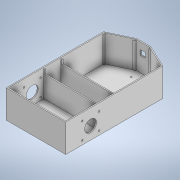
# Autodesk Inventor part: Robot
Saved by Autodesk Inventor 2020 (Build 240168000, 168)
## iProperties
Created: 2020-03-26
Part Number: Robot
Material: Generic
Document SubType Name: Modeling
Designer: Ondra
Density: 1 g/cm^3
Appearance: Default
Author: Ondra
Autodesk Inventor part; units mm, degrees
ref_plane "YZ Plane" through (0, 0, 0) normal (1, 0, 0) x (0, 1, 0)
ref_plane "XZ Plane" through (0, 0, 0) normal (0, 1, 0) x (-1, 0, 0)
ref_plane "XY Plane" through (0, 0, 0) normal (0, 0, 1) x (1, 0, 0)
sketch "Sketch1" plane through (0, 0, 0) normal (0, 1, 0) x (-1, 0, 0)
  line L0 (0, 0) -> (110, 0)
  line L1 (110, 0) -> (110, -180)
  line L2 (0, -180) -> (0, 0)
  line L3 (67.5, -200) -> (42.5, -200)
  line L4 (67.5, -200) -> (110, -180)
  line L5 (42.5, -200) -> (0, -180)
  dimension "d2" = 180
  dimension "d38" = 25
  constraints: 12 end point, 1 horizontal, 1 parallel, 1 perpendicular
  measures "d2" distance of L0.end L1.end
  measures "d38" distance of L3.start L3.end
extrude "Extrusion1" add sketch "Sketch1" along normal blind 2
sketch "Sketch2" plane through (0, 2, 0) normal (0, 1, 0) x (1, 0, 0)
  line L0 (0, 180) -> (-110, 180) projected
  line L1 (-110, 180) -> (-110, 0) projected
  line L2 (0, 180) -> (-110, 180)
  line L3 (-110, 180) -> (-110, 0)
  line L4 (-110, 0) -> (0, 0)
  line L5 (0, 0) -> (0, 180)
  line L6 (0, 0) -> (0, 180) projected
  line L7 (-110, 0) -> (0, 0) projected
  line L8 (-2, 2) -> (-108, 2)
  line L9 (-108, 2) -> (-108, 178)
  line L10 (-108, 178) -> (-2, 178)
  line L11 (-2, 178) -> (-2, 2)
  constraints: 16 end point, 4 parallel, 2 horizontal, 2 perpendicular
extrude "Extrusion2" add sketch "Sketch2" along normal blind 50
sketch "Sketch3" plane through (-108, 2, -2) normal (1, 0, 0) x (0, 0, -1)
  line L0 (0, 50) -> (176, 50) projected
  line L1 (65, 40) -> (65, 0)
  line L2 (176, 0) -> (0, 0) projected
  line L3 (67, 40) -> (67, 0)
  line L4 (67, 0) -> (65, 0)
  line L5 (97, 40) -> (97, 0)
  line L6 (97, 0) -> (99, 0)
  line L7 (99, 0) -> (99, 40)
  line L8 (65, 40) -> (67, 40)
  line L9 (99, 40) -> (97, 40)
  point P0 (-2, -2)
  point P1 (67, 0)
  constraints: 16 end point, 5 point on line, 4 perpendicular
extrude "Extrusion3" add sketch "Sketch3" along normal up to next
sketch "Sketch4" plane through (0, 2, 0) normal (0, 1, 0) x (1, 0, 0)
  line L0 (-108, 69) -> (-2, 69) projected
  line L1 (-90, 69) -> (-90, 99)
  line L2 (-108, 99) -> (-2, 99) projected
  line L3 (-2, 69) -> (-2, 99) projected
  line L4 (-20, 69) -> (-20, 99)
  line L5 (-20, 99) -> (-90, 99)
  line L6 (-90, 69) -> (-20, 69)
  point P0 (0, 0)
  constraints: 8 end point, 2 point on line, 1 collinear, 1 perpendicular
extrude "Extrusion4" cut sketch "Sketch4" against normal up to next contours L1 L2 L4 L0
sketch "Sketch5" plane through (-108, 2, -178) normal (1, 0, 0) x (0, 0, -1)
  line L0 (-111, 0) -> (-111, 40) projected
  line L1 (-111, 0) -> (-176, 0) projected
  circle A0 centre (-132, 21) radius 11
  circle A1 centre (-147.5, 36.5) radius 1.5
  circle A2 centre (-116.5, 36.5) radius 1.5
  circle A3 centre (-147.5, 36.5) radius 1.5
  circle A4 centre (-147.5, 5.5) radius 1.5
  circle A5 centre (-116.5, 5.5) radius 1.5
  point P0 (-178, -2)
  constraints: 6 centre point
extrude "Extrusion5" cut sketch "Sketch5" along normal through all both and the other way through all
sketch "Sketch6" plane through (-108, 2, -178) normal (0, 0, 1) x (1, 0, 0)
  line L0 (106, 0) -> (106, 50) projected
  line L1 (106, 50) -> (0, 50)
  line L2 (0, 50) -> (0, 0)
  line L3 (0, 0) -> (106, 0)
  line L4 (106, 0) -> (106, 50)
  point P0 (108, -2)
  constraints: 8 end point, 2 parallel, 1 horizontal, 1 perpendicular
extrude "Extrusion6" cut sketch "Sketch6" against normal up to next
sketch "Sketch7" plane through (0, 2, 0) normal (0, 1, 0) x (1, 0, 0)
  line L0 (-67.5, 200) -> (-110, 180) projected
  line L1 (-110, 180) -> (-67.5, 200)
  line L2 (-67.5, 200) -> (-42.5, 200)
  line L3 (0, 180) -> (-42.5, 200) projected
  line L4 (-42.5, 200) -> (0, 180)
  line L5 (-67.5, 198) -> (-42.5, 198)
  line L6 (-99.9511, 182.7289) -> (-67.5, 198)
  line L7 (-99.9511, 182.7289) -> (-108, 178.9412)
  line L8 (-108, 180) -> (-108, 101) projected
  line L9 (-108, 180) -> (-110, 180)
  line L10 (-21.25, 188) -> (-42.5, 198)
  line L11 (-21.25, 188) -> (-2, 178.9412)
  line L12 (-2, 101) -> (-2, 180) projected
  line L13 (-2, 180) -> (0, 180)
  line L14 (0, 180) -> (-42.5, 200)
  line L15 (-42.5, 200) -> (-67.5, 200) projected
  line L16 (-42.5, 200) -> (-67.5, 200)
  line L17 (-110, 180) -> (-110, 0) projected
  line L18 (-67.5, 200) -> (-110, 180)
  point P0 (0, 0)
  constraints: 26 end point, 4 point on line, 3 collinear, 1 horizontal, 1 parallel, 1 perpendicular
extrude "Extrusion7" add sketch "Sketch7" along normal up to surface (50 mm away)
sketch "Sketch8" plane through (-42.5, 0, -200) normal (0, 0, -1) x (-1, 0, 0)
  line L0 (0, 0) -> (25, 0) projected
  line L1 (8, 39.5) -> (17, 39.5)
  line L2 (17, 39.5) -> (17, 30.5)
  line L3 (17, 30.5) -> (8, 30.5)
  line L4 (8, 30.5) -> (8, 39.5)
  line L5 (8, 39.5) -> (17, 30.5) construction
  line L6 (17, 39.5) -> (8, 30.5) construction
  point P0 (-42.5, 0)
  dimension "d48" = 9
  dimension "d49" = 9
  constraints: 12 end point, 2 parallel, 1 horizontal, 1 perpendicular
  measures "d48" distance of L2.end L3.end
  measures "d49" distance of L1.end L2.end
extrude "Extrusion8" cut sketch "Sketch8" against normal blind 2
sketch "Sketch9" plane through (0, 2, 0) normal (0, 1, 0) x (1, 0, 0)
  line L0 (-108, 2) -> (-108, 178.9412) projected
  line L1 (-108, 2) -> (-106, 2)
  line L2 (-106, 2) -> (-106, 4)
  line L3 (-106, 4) -> (-108, 4)
  line L4 (-108, 4) -> (-108, 2)
  line L5 (-2, 2) -> (-108, 2) projected
  line L6 (-2, 2) -> (-4, 2)
  line L7 (-4, 2) -> (-4, 4)
  line L8 (-4, 4) -> (-2, 4)
  line L9 (-2, 4) -> (-2, 2)
  line L10 (-67.5, 198) -> (-108, 178.9412) projected
  line L11 (-106, 178.9412) -> (-106, 176.9412)
  line L12 (-106, 176.9412) -> (-108, 176.9412)
  line L13 (-108, 176.9412) -> (-108, 178.9412)
  line L14 (-106, 178.9412) -> (-106, 179.8824)
  line L15 (-108, 178.9412) -> (-108, 101) projected
  line L16 (-108, 178.9412) -> (-106, 179.8824)
  line L17 (-2, 178.9412) -> (-2, 2) projected
  line L18 (-4, 178.9412) -> (-4, 176.9412)
  line L19 (-4, 176.9412) -> (-2, 176.9412)
  line L20 (-2, 176.9412) -> (-2, 178.9412)
  line L21 (-4, 178.9412) -> (-4, 179.8824)
  line L22 (-2, 178.9412) -> (-42.5, 198) projected
  line L23 (-4, 179.8824) -> (-2, 178.9412)
  line L24 (-4, 179.8824) -> (-2, 178.9412)
  line L25 (-67.5, 198) -> (-108, 178.9412) projected
  line L26 (-67.5, 198) -> (-67.5, 196)
  line L27 (-67.5, 196) -> (-71.75, 196)
  line L28 (-42.5, 198) -> (-67.5, 198) projected
  line L29 (-42.5, 198) -> (-42.5, 196)
  line L30 (-42.5, 196) -> (-38.25, 196)
  line L31 (-42.5, 198) -> (-38.25, 196)
  line L32 (-71.75, 196) -> (-67.5, 198)
  line L33 (-55, 2) -> (-53, 2)
  line L34 (-53, 2) -> (-53, 4)
  line L35 (-53, 4) -> (-57, 4)
  line L36 (-57, 4) -> (-57, 2)
  line L37 (-57, 2) -> (-55, 2)
  point P0 (0, 0)
  constraints: 60 end point, 7 point on line, 6 parallel, 5 perpendicular, 3 collinear, 3 vertical, 2 horizontal, 1 midpoint
extrude "Extrusion9" add sketch "Sketch9" along normal blind 48 contours L0 L3 L2 L1 | L36 L35 L34 L5 | L0 L10 L14 L11 L12 | L7 L8 L9 L5 | L10 L26 L27 | L22 L30 L29 | L19 L18 L21 L22 L17
sketch "Sketch10" plane through (-108, 42, -101) normal (0, 1, 0) x (1, 0, 0)
  line L0 (0, 0) -> (106, 0) projected
  line L1 (0, -2) -> (106, -2) projected
  line L2 (106, 0) -> (104, 0)
  line L3 (104, 0) -> (104, -2)
  line L4 (104, -2) -> (106, -2)
  line L5 (106, -2) -> (106, 0)
  line L6 (106, -32) -> (106, -34) projected
  line L7 (106, -32) -> (104, -32)
  line L8 (104, -32) -> (104, -34)
  line L9 (104, -34) -> (106, -34)
  line L10 (106, -34) -> (106, -32)
  line L11 (106, -34) -> (0, -34) projected
  line L12 (0, -32) -> (18, -32) projected
  line L13 (0, -34) -> (2, -34)
  line L14 (2, -34) -> (2, -32)
  line L15 (2, -32) -> (0, -32)
  line L16 (0, -32) -> (0, -34)
  line L17 (0, -2) -> (0, 0) projected
  line L18 (0, 0) -> (2, 0)
  line L19 (2, 0) -> (2, -2)
  line L20 (2, -2) -> (0, -2)
  line L21 (0, -2) -> (0, 0)
  point P0 (108, -101)
  point P1 (2, -34)
  point P2 (2, -2)
  point P3 (2, 0)
  constraints: 32 end point, 8 parallel, 4 horizontal, 4 perpendicular, 3 point on line
extrude "Extrusion10" add sketch "Sketch10" along normal blind 8 contours L0 L19 L1 L17 | L0 L5 L1 L3 | L11 L16 L12 L14 | L6 L9 L8 L7
sketch "Sketch12" plane through (0, 2, 0) normal (0, 1, 0) x (1, 0, 0)
  line L0 (-106, 99) -> (-4, 99) projected
  line L1 (-55, 99) -> (-100, 99)
  line L2 (-100, 99) -> (-100, 69)
  line L3 (-108, 101) -> (-2, 101) projected
  line L4 (-100, 99) -> (-70, 99) construction
  line L5 (-108, 99) -> (-108, 69) projected
  line L6 (-108, 99) -> (-100, 99)
  line L7 (-100, 99) -> (-100, 69)
  line L8 (-100, 69) -> (-108, 69)
  line L9 (-108, 69) -> (-108, 99)
  line L10 (-10, 99) -> (-10, 69)
  line L11 (-2, 99) -> (-2, 69)
  line L12 (-2, 99) -> (-10, 99)
  line L13 (-10, 99) -> (-10, 69)
  line L14 (-10, 69) -> (-2, 69)
  line L15 (-2, 69) -> (-2, 99)
  point P0 (0, 0)
  constraints: 26 end point, 3 perpendicular, 2 horizontal, 2 parallel, 1 midpoint, 1 point on line
extrude "Extrusion12" add sketch "Sketch12" along normal blind 6
sketch "Sketch13" plane through (0, 2, 0) normal (0, 1, 0) x (1, 0, 0)
  line L0 (-42.5, 198) -> (-67.5, 198) projected
  circle A0 centre (-61.75, 183) radius 1.5
  circle A1 centre (-48.25, 183) radius 1.5
  point P0 (0, 0)
  constraints: 2 centre point
extrude "Extrusion13" cut sketch "Sketch13" against normal through all
body "Solid1"
